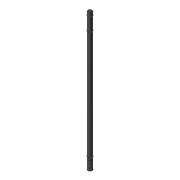
# Autodesk Inventor part: vailla enroscada
Saved by Autodesk Inventor 2022 (Build 260153000, 153)
## iProperties
Created: 2019-06-18
Part Number: vailla enroscada
Material: Acetal Resin, Black
Document SubType Name: Modeling
Designer: usuario_2
Density: 1.425 g/cm^3
Appearance: Smooth - Black
Author: usuario_2
Autodesk Inventor part; units mm, degrees
ref_plane "YZ Plane" through (0, 0, 0) normal (1, 0, 0) x (0, 1, 0)
ref_plane "XZ Plane" through (0, 0, 0) normal (0, 1, 0) x (-1, 0, 0)
ref_plane "XY Plane" through (0, 0, 0) normal (0, 0, 1) x (1, 0, 0)
sketch "Boceto1" plane through (0, 0, 0) normal (0, 0, 1) x (1, 0, 0)
  circle A0 centre (0, 0) radius 5
  dimension "d0" = 5
  constraints: 1 centre point, 1 coincident
  measures "d0" radius of A0
extrude "Extrusión1" add sketch "Boceto1" along normal blind 310
thread "Rosca1" size "M10x1.5" class "6g" standard "ANSI Metric M Profile" length 20
fillet "Empalme1" radius 2 1 edges at (-5, 0, 310)
sketch "Boceto2" plane through (0, 0, 0) normal (0, 1, 0) x (-1, 0, 0)
  line L0 (-3, 310) -> (3, 310) construction
  line L1 (0, 310) -> (0, 0) construction
  line L2 (-5, 0) -> (-5, 308) construction
  line L3 (5, 0) -> (5, 308) projected
  line L4 (5, 300) -> (4, 300)
  line L5 (4, 300) -> (4, 301.5)
  line L6 (4, 301.5) -> (5, 301.5)
  line L7 (5, 301.5) -> (5, 300)
  line L8 (5, 0) -> (5, 308) projected
  line L9 (5, 26.5) -> (4, 26.5)
  line L10 (4, 26.5) -> (4, 25)
  line L11 (4, 25) -> (5, 25)
  line L12 (5, 25) -> (5, 26.5)
  line L13 (-5, 0) -> (5, 0) projected
  line L14 (5, 272) -> (4, 272)
  line L15 (4, 272) -> (4, 270.5)
  line L16 (4, 270.5) -> (5, 270.5)
  line L17 (5, 270.5) -> (5, 272)
  dimension "d6" = 1.5
  dimension "d7" = 1
  dimension "d9" = 10
  dimension "d11" = 25
  dimension "d12" = 1.5
  dimension "d13" = 1
  dimension "d14" = 1.5
  dimension "d15" = 1
  dimension "d16" = 39.5
  constraints: 26 end point, 7 parallel, 3 horizontal, 3 perpendicular, 3 point on line, 1 midpoint
  measures "d6" distance of L4.end L5.end
  measures "d7" distance of L5.end L6.end
  measures "d9" distance between parallel lines of L0 L4
  measures "d11" distance between parallel lines of L13 L11
  measures "d12" distance of L9.end L10.end
  measures "d13" distance of L9.start L9.end
  measures "d14" distance of L14.end L15.end
  measures "d15" distance of L14.start L14.end
  measures "d16" distance between parallel lines of L0 L16
revolve "Revolución1" cut sketch "Boceto2" angle 360 about axis through (0, 0, 310) along (0, 0, -1)
